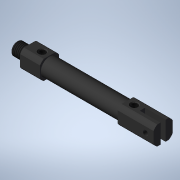
# Autodesk Inventor part: CJ2D10-25Z(1_0)_BODY
Saved by Autodesk Inventor 2021 (Build 250183000, 183)
## iProperties
Created: 2025-12-08
Part Number: CJ2D10-25Z(1_0)_BODY
Material: Generic
Catalog Web Link: www.3dfindit.com
Description: CJ2-Z BODY-Air Cylinder/Standard: Double Acting Single Rod
Vendor: SMC
Document SubType Name: Modeling
Designer: psAdmin
Manufacturer: SMC
Mass: 6.4376 g
Surface Area: 54.3155 cm^2
Volume: 6.4376 cm^3
Density: 1 g/cm^3
Appearance: PSOLRGB-176-176-176
Category: PARTsolutions
Company: SMC
Title: CJ2D10-25Z_BODY
Author: Cadenas PARTsolutions
Comments: Air Cylinder/Standard: Double Acting Single Rod
PSOL_IDENT_0: {$CADENAS_DATA/23d-libs/smc_jp/actuator/standard_air_cylinder/cj2/cj2_z/parts/cj2_z_body.prj},261 {V
PSOL_IDENT_1: TYP=3D},{NB=CJ2D10-25Z(1_0)_BODY},{LINA=CJ2D10-25Z_BODY},{NN=CJ2-Z BODY},{DATE=02.12.2025 09:45:30},
PSOL_IDENT_2: {GEOMDATE=23.08.2024 09:13:24},{VERSION=},{LINEID=390},{WBVAR=AUTOSWITCH,NUMBER,CUSHION,STOP,STROKE,
PSOL_IDENT_3: PORT,MOUNTING,OMSCXC3,OMSCXC51,THREAD},{WBNUMERIC=STROKE}  {NB=CJ2D10-25Z(1_0)_BODY},{LINA=CJ2D10-25
PSOL_IDENT_4: Z_BODY},{KT=DUMMY},{ORDER=CJ2D10-25Z},{BORE=10},{MOUNT=(D) Double clevis},{AUTOSWITCH=},{NUMBER=},{C
PSOL_IDENT_5: USHION=},{MOUNTX=D},{STOP=1},{STROKE=25},{SMAX=400},{PORT=},{MOUNTING=},{OMSCXC3=},{OMSCXC51=},{THRE
PSOL_IDENT_6: AD=0},{B=12.0},{B1X1=12.0},{B2=15.000},{C=14},{C1X1=14.0},{C2=17.000},{CD=3.3},{U=8},{CX=3.2},{CZ=0}
PSOL_IDENT_7: ,{CZ1X1=0.0},{D=4},{F=8},{GA=8.0},{GA1X1=8.0},{GA2=7.500},{GB=18.0},{GB1X1=18.0},{GB2=19.500},{H=28}
PSOL_IDENT_8: ,{NA=12.5},{NA1X1=12.5},{NA2=21.000},{NB1=22.5},{NB1X1=22.5},{NB2=33.000},{NDH8=-},{NDH81=0},{NN=M8x
PSOL_IDENT_9: 1.0},{NN1=8},{NN2=1.0},{R=5},{S=46},{S1X1=46.0},{S2X2=65.000},{WA=14.5},{WB=13.5},{WW=4.5},{MOUNTING
PSOL_IDENT_10: X='','(-) None','-A','(A) Rail mounting','-B','(B) Band mounting'},{PORTX='', '(-) Perpendicular'},{
PSOL_IDENT_11: SWX=4.5},{SW1=6.000},{SW2=2.000},{SW3=2.500},{SW4=1.500},{SW5=4.500},{SW6=0.500},{SW7=3.000},{SW8=3.
PSOL_IDENT_12: 500},{SW9=0.500},{SW=4.5},{SWSINX= '','N/A' },{NENN=CJ2D10},{X1=6.000},{X2=7.750},{Y1=2.300},{Y2=6.7
PSOL_IDENT_13: 50},{X=6},{Y=2.3},{XC3= '','(-) None','-XC3AB','(XC3AB) Rod port location viewed: A,Head port locati
PSOL_IDENT_14: on viewed: B','-XC3AC','(XC3AC) Rod port location viewed: A,Head port location viewed: C','-XC3AD','
PSOL_IDENT_15: (XC3AD) Rod port location viewed: A,Head port location viewed: D','-XC3BA','(XC3BA) Rod port locatio
PSOL_IDENT_16: n viewed: B,Head port location viewed: A','-XC3BB','(XC3BB) Rod port location viewed: B,Head port lo
PSOL_IDENT_17: cation viewed: B','-XC3BC','(XC3BC) Rod port location viewed: B,Head port location viewed: C','-XC3B
PSOL_IDENT_18: D','(XC3BD) Rod port location viewed: B,Head port location viewed:D','-XC3CA','(XC3CA) Rod port loca
PSOL_IDENT_19: tion viewed: C,Head port location viewed: A','-XC3CB','(XC3CB) Rod port location viewed: C,Head port
PSOL_IDENT_20: location viewed: B','-XC3CC','(XC3CC) Rod port location viewed: C,Head port location viewed: C','-X
PSOL_IDENT_21: C3CD','(XC3CD) Rod port location viewed: C,Head port location viewed:D','-XC3DA','(XC3DA) Rod port l
PSOL_IDENT_22: ocation viewed: D,Head port location viewed: A','-XC3DB','(XC3DB) Rod port location viewed: D,Head p
PSOL_IDENT_23: ort location viewed: B','-XC3DC','(XC3DC) Rod port location viewed: D,Head port location viewed: C','
PSOL_IDENT_24: -XC3DD','(XC3DD) Rod port location viewed: D,Head port location viewed:D' },{PORTXC3=A1},{PORTXC32=A
PSOL_IDENT_25: 2},{CUSHIONX= '','(-) Rubber cushion','A','(A) Air cushion' },{XC51= '','(-) None','-XC51H4','(XC51H
PSOL_IDENT_26: 4) Hose nipple type: ø4/2.5 with restriction','-XC51H6','(XC51H6) Hose nipple type: ø6/4 with restri
PSOL_IDENT_27: ction','-XC51MH4','(XC51MH4) Hose nipple type: ø4/2.5 without restriction','-XC51MH6','(XC51MH6) Hos
PSOL_IDENT_28: e nipple type: ø6/4 without restriction' },{MODEL=M-5H-6},{PINMODEL=CD-J010},{SWAB=3.5},{SWABD=0}
NB: CJ2D10-25Z(1_0)_BODY
NN: M8x1.0
NT: Air Cylinder/Standard: Double Acting Single Rod
NBSYN: $ORDER.($STOP._$THREAD.)_BODY
LINA: CJ2D10-25Z_BODY
CATALOG: SMC (JP
ROWDESC: CJ2D10
BORE: 10
MOUNT: (D) Double clevis
AUTOSWITCH: (-) Without autoswitch
NUMBER: N/A
CUSHION: (-) Rubber cushion
STOP: Manufacturable stroke
STROKE: 25
SMAX: 400
PORT: (-) Perpendicular
MOUNTING: (-) None
OMSCXC3: (-) None
OMSCXC51: (-) None
THREAD: on
B: 12
B1X1: 12
B2: 15
C: 14
C1X1: 14
C2: 17
CD: 3.3
U: 8
CX: 3.2
CZ: 0
CZ1X1: 0
D: 4
F: 8
GA: 8
GA1X1: 8
GA2: 7.5
GB: 18
GB1X1: 18
GB2: 19.5
H: 28
NA: 12.5
NA1X1: 12.5
NA2: 21
NB1: 22.5
NB1X1: 22.5
NB2: 33
NDH8: -
NDH81: 0
NN1: 8
NN2: 1
R: 5
S: 46
S1X1: 46
S2X2: 65
WA: 14.5
WB: 13.5
WW: 4.5
SW1: 6
SW2: 2
SW3: 2.5
SW4: 1.5
SW5: 4.5
SW6: 0.5
SW7: 3
SW8: 3.5
SW9: 0.5
X1: 6
X2: 7.75
Y1: 2.3
Y2: 6.75
SUPPLIER: SMC
ARTICLENO: CJ2D10-25Z(1_0)_BODY
BOMINFO: CJ2D10-25Z_BODY
CREATOR: CADENAS GmbH
Autodesk Inventor part; units mm, degrees
sketch "Sketch_8" plane through (0, 0, 0) normal (0, 0, 1) x (1, 0, 0)
  line L0 (0, 0) -> (-8, 0)
  line L1 (-8, 0) -> (-8, 3.3865)
  line L2 (-8, 3.3865) -> (-7.3865, 4)
  line L3 (-7.3865, 4) -> (0, 4)
  line L4 (0, 4) -> (0, 0)
  line L5 (0, 0) -> (-8, 0)
  constraints: 12 end point
revolve "Revolution1" add sketch "Sketch_8" angle 360 about axis through (0, 0, 0) along (1, 0, 0)
thread "Thread1" size "M8x1" class "6g" standard "ISO Metric profile" length 5.8865
sketch "Sketch_9" plane through (0, 0, 0) normal (1, 0, 0) x (0, 0, -1)
  line L0 (-6, 3.6056) -> (-6, -3.6056)
  arc A0 (-6, -3.6056) -> (-3.6056, -6) centre (0, 0) ccw
  line L1 (-3.6056, -6) -> (3.6056, -6)
  arc A1 (3.6056, -6) -> (6, -3.6056) centre (0, 0) ccw
  line L2 (6, -3.6056) -> (6, 3.6056)
  arc A2 (6, 3.6056) -> (3.6056, 6) centre (0, 0) ccw
  line L3 (3.6056, 6) -> (-3.6056, 6)
  arc A3 (-3.6056, 6) -> (-6, 3.6056) centre (0, 0) ccw
  constraints: 8 end point, 8 point on circle, 4 centre point
extrude "Extrusion1" add sketch "Sketch_9" along normal blind 12.5
sketch "Sketch_6" plane through (12.5, 0, 0) normal (1, 0, 0) x (0, 0, -1)
  circle A0 centre (0, 0) radius 5.5
  constraints: 1 centre point
extrude "Extrusion2" add sketch "Sketch_6" along normal blind 49
sketch "Sketch_10" plane through (61.5, 0, 0) normal (1, 0, 0) x (0, 0, -1)
  line L0 (-6, 3.6056) -> (-6, -3.6056)
  arc A0 (-6, -3.6056) -> (-3.6056, -6) centre (0, 0) ccw
  line L1 (-3.6056, -6) -> (3.6056, -6)
  arc A1 (3.6056, -6) -> (6, -3.6056) centre (0, 0) ccw
  line L2 (6, -3.6056) -> (6, 3.6056)
  arc A2 (6, 3.6056) -> (3.6056, 6) centre (0, 0) ccw
  line L3 (3.6056, 6) -> (-3.6056, 6)
  arc A3 (-3.6056, 6) -> (-6, 3.6056) centre (0, 0) ccw
  constraints: 8 end point, 8 point on circle, 4 centre point
extrude "Extrusion3" add sketch "Sketch_10" along normal blind 22.5
sketch "Sketch7" plane through (0, 0, 0) normal (0, 0, 1) x (1, 0, 0)
  line L0 (8, 6) -> (8, 1)
  line L1 (8, -0.1934) -> (5.933, 1)
  line L2 (5.933, 1) -> (5.933, 5.567)
  line L3 (5.933, 5.567) -> (5.5, 6)
  line L4 (5.5, 6) -> (8, 6)
  line L5 (8, 6) -> (8, -0.1934)
  constraints: 12 end point
revolve "Revolution2" cut sketch "Sketch7" angle 360 about axis through (8, 6, 0) along (0, 1, 0)
thread "Thread2" size "M5x0.8" class "6H" standard "ISO Metric profile" full length
sketch "Sketch_7" plane through (0, 0, 0) normal (0, 0, 1) x (1, 0, 0)
  line L0 (66, 6) -> (66, 1)
  line L1 (66, -0.1934) -> (63.933, 1)
  line L2 (63.933, 1) -> (63.933, 5.567)
  line L3 (63.933, 5.567) -> (63.5, 6)
  line L4 (63.5, 6) -> (66, 6)
  line L5 (66, 6) -> (66, -0.1934)
  constraints: 12 end point
revolve "Revolution3" cut sketch "Sketch_7" angle 360 about axis through (66, 6, 0) along (0, 1, 0)
thread "Thread3" size "M5x0.8" class "6H" standard "ISO Metric profile" full length
sketch "Sketch_16" plane through (0, 0, 0) normal (0, 0, 1) x (1, 0, 0)
  line L0 (42.5, 0) -> (-8, 0)
  line L1 (-8, 0) -> (-8, 2)
  line L2 (-8, 2) -> (12.5, 2)
  line L3 (12.5, 2) -> (12.5, 5)
  line L4 (12.5, 5) -> (42.5, 5)
  line L5 (42.5, 5) -> (42.5, 0)
  line L6 (42.5, 0) -> (-8, 0)
  constraints: 14 end point
revolve "Revolution4" cut sketch "Sketch_16" angle 360 about axis through (42.5, 0, 0) along (1, 0, 0)
sketch "Sketch_3" plane through (0, 0, 0) normal (0, 1, 0) x (-1, 0, 0)
  line L0 (-71, 1.6) -> (-84, 1.6)
  line L1 (-84, 1.6) -> (-84, -1.6)
  line L2 (-84, -1.6) -> (-71, -1.6)
  line L3 (-71, -1.6) -> (-71, 1.6)
  constraints: 8 end point
extrude "Extrusion4" cut sketch "Sketch_3" along normal mid plane 12
sketch "Sketch_13" plane through (0, 0, 0) normal (0, 0, 1) x (1, 0, 0)
  circle A0 centre (79, 0) radius 1.65
  constraints: 1 centre point
extrude "Extrusion5" cut sketch "Sketch_13" along normal mid plane 12
ref_plane "BODY_N_XY" through (79, 0, 0) normal (0, 0, -1) x (1, 0, 0)
ref_plane "BODY_N_YZ" through (79, 0, 0) normal (1, 0, 0) x (0, -1, 0)
ref_plane "BODY_N_ZX" through (79, 0, 0) normal (0, -1, 0) x (0, 0, -1)
ref_plane "BODY_PIN_XY" through (79, 0, 0) normal (-1, 0, 0) x (0, 0, -1)
ref_plane "BODY_PIN_YZ" through (79, 0, 0) normal (0, 0, -1) x (0, -1, 0)
ref_plane "BODY_PIN_ZX" through (79, 0, 0) normal (0, -1, 0) x (-1, 0, 0)
ref_plane "NUT2_XY" through (71, 0, 0) normal (1, 0, 0) x (0, 0, -1)
ref_plane "NUT2_YZ" through (71, 0, 0) normal (0, 0, -1) x (0, 1, 0)
ref_plane "NUT2_ZX" through (71, 0, 0) normal (0, 1, 0) x (1, 0, 0)
ref_plane "SW1_XY" through (17, 0, 0) normal (1, 0, 0) x (0, 0, -1)
ref_plane "SW1_YZ" through (17, 0, 0) normal (0, 0, -1) x (0, 1, 0)
ref_plane "SW1_ZX" through (17, 0, 0) normal (0, 1, 0) x (1, 0, 0)
ref_plane "SW2_XY" through (57, 0, 0) normal (-1, 0, 0) x (0, 0, -1)
ref_plane "SW2_YZ" through (57, 0, 0) normal (0, 0, -1) x (0, -1, 0)
ref_plane "SW2_ZX" through (57, 0, 0) normal (0, -1, 0) x (-1, 0, 0)
ref_plane "SW_R1_XY" through (17, -11, 0) normal (1, 0, 0) x (0, 0, -1)
ref_plane "SW_R1_YZ" through (17, -11, 0) normal (0, 0, -1) x (0, 1, 0)
ref_plane "SW_R1_ZX" through (17, -11, 0) normal (0, 1, 0) x (1, 0, 0)
ref_plane "SW_R2_XY" through (57, -11, 0) normal (-1, 0, 0) x (0, 0, -1)
ref_plane "SW_R2_YZ" through (57, -11, 0) normal (0, 0, -1) x (0, -1, 0)
ref_plane "SW_R2_ZX" through (57, -11, 0) normal (0, -1, 0) x (-1, 0, 0)
ref_plane "body_XY" through (0, 0, 0) normal (-1, 0, 0) x (0, 0, -1)
ref_plane "body_YZ" through (0, 0, 0) normal (0, 0, -1) x (0, -1, 0)
ref_plane "body_ZX" through (0, 0, 0) normal (0, -1, 0) x (-1, 0, 0)
body "Solid1"
